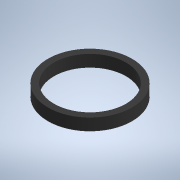
# Autodesk Inventor part: 6138k63_seal
Saved by Autodesk Inventor 2020.1 (Build 241239000, 239)
## iProperties
Created: 2019-10-27
Part Number: 6138k63_seal
Material: Rubber, Silicone
Document SubType Name: Modeling
Designer: agmle
Mass: 0.0118153 g
Surface Area: 0.581908 cm^2
Volume: 0.00945224 cm^3
Density: 1.25 g/cm^3
Appearance: Rubber - Black
Author: agmle
Autodesk Inventor part; units mm, degrees
ref_plane "YZ Plane" through (0, 0, 0) normal (1, 0, 0) x (0, 1, 0)
ref_plane "XZ Plane" through (0, 0, 0) normal (0, 1, 0) x (-1, 0, 0)
ref_plane "XY Plane" through (0, 0, 0) normal (0, 0, 1) x (1, 0, 0)
sketch "Sketch1" plane through (0, 0, 0) normal (0, 0, 1) x (1, 0, 0)
  line L0 (2.9308, 0.485) -> (3.4192, 0.485)
  line L1 (3.4192, 0.485) -> (3.4192, -0.485)
  line L2 (3.4192, -0.485) -> (2.9308, -0.485)
  line L3 (2.9308, -0.485) -> (2.9308, 0.485)
  line L4 (0, 0) -> (2.9308, 0) construction
  line L5 (0, -0.679) -> (0, 0.679) projected
  dimension "d0" = 0.4885
  dimension "d1" = 0.97
  dimension "d2" = 2.9308
  constraints: 10 end point, 2 horizontal, 2 parallel, 1 midpoint, 1 perpendicular
  measures "d0" distance of L0.start L0.end
  measures "d1" distance of L0.end L1.end
  measures "d2" distance from line of L4.start L3
revolve "Revolution1" add sketch "Sketch1" angle 360 about axis through (0, -10, 0) along (0, 1, 0)
body "Solid1"
